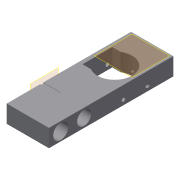
# Autodesk Inventor part: 01_Slide_camera_x_v0
Saved by Autodesk Inventor 2019.4 (Build 234330000, 330)
## iProperties
Created: 2020-10-27
Part Number: 01_Slide_camera_x_v0
Material: Generic
Document SubType Name: Modeling
Designer: diederichbenedict
Density: 1 g/cm^3
Appearance: Default
Author: diederichbenedict
Autodesk Inventor part; units mm, degrees
ref_plane "YZ Plane" through (0, 0, 0) normal (1, 0, 0) x (0, 1, 0)
ref_plane "XZ Plane" through (0, 0, 0) normal (0, 1, 0) x (-1, 0, 0)
ref_plane "XY Plane" through (0, 0, 0) normal (0, 0, 1) x (1, 0, 0)
ref_plane "Work Plane1" through (49.1675, 65.1721, -19.9847) normal (0, 1, 0) x (-1, 0, 0)
sketch "Sketch1" plane through (49.1675, 65.1721, -19.9847) normal (0, 1, 0) x (-1, 0, 0)
  circle A0 centre (-2.8102, 4.1616) radius 0.75 construction
  circle A1 centre (-2.8102, 25.1616) radius 0.75 construction
  line L0 (11.6898, 12.5705) -> (11.6898, 16.7526) construction
  arc A2 (11.6898, 16.7526) -> (11.6898, 12.5705) centre (-2.8102, 14.6616) ccw construction
  arc A3 (6.4943, 19.8433) -> (3.1979, 23.455) centre (-2.8102, 14.6616) ccw construction
  arc A4 (3.1979, 5.8681) -> (6.3691, 9.2612) centre (-2.8102, 14.6616) ccw construction
  line L1 (6.4943, 19.8433) -> (10.0762, 19.8433) construction
  line L2 (10.0762, 19.8433) -> (10.0762, 9.2612) construction
  line L3 (10.0762, 9.2612) -> (6.3691, 9.2612) construction
  arc A5 (-8.8183, 23.455) -> (-8.8183, 5.8681) centre (-2.8102, 14.6616) ccw construction
  line L4 (15.1898, -17.3384) -> (-20.8102, -17.3384)
  line L5 (-20.8102, -17.3384) -> (-20.8102, 14.6616)
  line L6 (-20.8102, 14.6616) -> (15.1898, 14.6616)
  line L7 (15.1898, 14.6616) -> (15.1898, -17.3384)
  arc A6 (4.8861, 27.3616) -> (3.5031, 1.2204) centre (-2.8102, 14.6616) ccw construction
  line L8 (4.8861, 27.3616) -> (11.8898, 27.3616) construction
  line L9 (11.8898, 27.3616) -> (11.8898, 1.9616) construction
  line L10 (11.8898, 1.9616) -> (4.7096, 1.9616) construction
  line L11 (4.7096, 1.9616) -> (2.6908, 5.7766) construction
  arc A7 (2.6908, 5.7766) -> (6.254, 9.4612) centre (-2.8102, 14.6616) ccw construction
  line L12 (6.254, 9.4612) -> (9.8762, 9.4612) construction
  line L13 (9.8762, 9.4612) -> (9.8762, 19.6433) construction
  line L14 (9.8762, 19.6433) -> (6.376, 19.6433) construction
  arc A8 (6.376, 19.6433) -> (3.2687, 23.1616) centre (-2.8102, 14.6616) ccw construction
  line L15 (3.2687, 23.1616) -> (-8.889, 23.1616) construction
  arc A9 (-8.889, 23.1616) -> (-8.446, 5.8616) centre (-2.8102, 14.6616) ccw construction
  line L16 (-8.446, 5.8616) -> (1.0472, 5.8616) construction
  line L17 (1.0472, 5.8616) -> (3.5031, 1.2204) construction
  arc A10 (-17.6602, 14.6616) -> (4.7096, 1.9616) centre (-2.9041, 14.6019) ccw
  line L18 (4.7096, 1.9616) -> (11.8943, 1.9616)
  line L19 (11.8943, 1.9616) -> (11.8898, 14.6616)
  line L20 (11.8898, 14.6616) -> (15.1898, 14.6616)
  line L21 (3.1979, 5.8681) -> (-8.8183, 5.8681) projected
  line L22 (3.1979, 23.455) -> (-8.8183, 23.455) projected
  point P0 (49.1675, 19.9847)
  dimension "d0" = 32
  dimension "d2" = 18
  dimension "d3" = 18
  dimension "d4" = 0.2
  constraints: 34 end point, 11 point on circle, 5 centre point, 2 midpoint, 2 parallel, 2 point on line, 1 collinear, 1 horizontal, 1 perpendicular, 4 other
  measures "d0" distance from line of L4 A6.centre
  measures "d2" distance from line of L7 A9.centre
  measures "d3" distance from line of L5 A6.centre
  measures "d4" radial gap between concentric circles of A2 A6
extrude "Extrusion1" add sketch "Sketch1" against normal blind 15 contours L4 L5 L6 A10 L18 L19 L7
mirror "Mirror1" about plane through (37.2777, 65.1721, -5.3231) normal (0, 0, 1) of "Extrusion1"
sketch "Sketch4" plane through (33.9777, 50.1721, -37.3231) normal (-1, 0, 0) x (0, 0, 1)
  line L0 (0, 15) -> (64, 15) projected
  line L1 (0, 15) -> (0, 0) projected
  line L2 (0, 0) -> (64, 0) projected
  line L3 (64, 15) -> (64, 0) projected
  line L4 (0, 15) -> (64, 15) projected
  line L5 (64, 15) -> (88, 15)
  line L6 (88, 15) -> (88, 0)
  line L7 (88, 0) -> (64, 0)
  line L8 (64, 0) -> (64, 15)
  circle A0 centre (56, 7.5) radius 3 projected
  circle A1 centre (56, 7.5) radius 5 projected
  circle A2 centre (76, 7.5) radius 6
  point P0 (37.3231, -50.1721)
  dimension "d20" = 24
  dimension "d21" = 12
  dimension "d24" = 12
  constraints: 8 end point, 2 parallel, 1 centre point, 1 horizontal, 1 perpendicular
  measures "d20" distance of L6.end L7.end
  measures "d21" diameter of A2
  measures "d24" distance from line of A2.centre L6
extrude "Extrusion4" add sketch "Sketch4" against normal up to surface (36 mm away) contours L5 L6 L7 L3
ref_plane "Work Plane4" through (33.9777, 57.6721, 36.6769) normal (1, 0, 0) x (0, 0, 1)
sketch "Sketch6" plane through (33.9777, 57.6721, 36.6769) normal (1, 0, 0) x (0, 0, 1)
  circle A0 centre (10, 0) radius 1.625 construction
  circle A1 centre (2, -8) radius 1.625 projected
  circle A2 centre (-6, 0) radius 1.625 construction
  circle A3 centre (2, 8) radius 1.625 projected
  circle A4 centre (2, 0) radius 4 projected
  circle A5 centre (2, 0) radius 11 construction
  line L0 (14, 7.5) -> (-74, 7.5) projected
  arc A6 (10.0467, 7.5) -> (-6.0467, 7.5) centre (2, 0) ccw
  point P0 (-36.6769, 57.6721)
  constraints: 4 point on circle, 2 point on line, 1 centre point, 1 concentric
extrude "Extrusion6" add sketch "Sketch6" along normal blind 15 contours A3 L0 | A3 L0 A6 | L0 A3
sketch "Sketch5" plane through (33.9777, 50.1721, -37.3231) normal (-1, 0, 0) x (0, 0, 1)
  circle A0 centre (68, 7.5) radius 1.625 projected
  circle A1 centre (84, 7.5) radius 1.625 projected
  circle A2 centre (84, 7.5) radius 1.45
  circle A3 centre (68, 7.5) radius 1.45
  circle A4 centre (76, 15.5) radius 1.625 projected
  circle A5 centre (76, -0.5) radius 1.625 projected
  circle A6 centre (76, -0.5) radius 1.45
  circle A7 centre (76, 15.5) radius 1.45
  point P0 (37.3231, -50.1721)
  dimension "d25" = 2.9
  dimension "d26" = 2.9
  dimension "d31" = 2.9
  dimension "d32" = 2.9
  constraints: 4 centre point, 4 coincident
  measures "d25" diameter of A2
  measures "d26" diameter of A3
  measures "d31" diameter of A6
  measures "d32" diameter of A7
extrude "Extrusion5" cut sketch "Sketch5" against normal blind 15 contours A2 | A3 | A6 | A7
sketch "Sketch7" plane through (33.9777, 50.1721, -37.3231) normal (-1, 0, 0) x (0, 0, 1)
  arc A0 (74.6389, 15) -> (77.3611, 15) centre (76, 15.5) ccw projected
  line L0 (0, 15) -> (74.6389, 15) projected
  line L1 (0, 15) -> (0, 0) projected
  line L2 (67.9533, 0) -> (0, 0) projected
  arc A1 (67.9533, 0) -> (84.0467, 0) centre (76, 7.5) ccw projected
  line L3 (88, 0) -> (84.0467, 0) projected
  line L4 (88, 15) -> (88, 0) projected
  line L5 (77.3611, 15) -> (88, 15) projected
  circle A2 centre (68, 7.5) radius 1.45 projected
  circle A3 centre (84, 7.5) radius 1.45 projected
  circle A4 centre (76, -0.5) radius 1.45 projected
  circle A5 centre (76, 7.5) radius 6 projected
  line L6 (0, 0) -> (88, 0) projected
  line L7 (88, 0) -> (106, 0)
  line L8 (106, 0) -> (106, 15)
  line L9 (106, 15) -> (88, 15)
  line L10 (88, 15) -> (88, 0)
  circle A6 centre (96, 7.5) radius 6.4305
  circle A7 centre (56, 7.5) radius 6.4532
  point P0 (37.3231, -50.1721)
  dimension "d34" = 20
  dimension "d35" = 10
  dimension "d40" = 20
  constraints: 8 end point, 2 centre point, 2 parallel, 1 horizontal, 1 perpendicular
  measures "d34" distance of A6.centre A1.centre
  measures "d35" distance from line of A6.centre L8
  measures "d40" distance of A1.centre A7.centre
extrude "Extrusion7" add sketch "Sketch7" against normal up to surface (36 mm away) contours L9 L8 L7 L4
sketch "Sketch9" plane through (33.9777, 50.1721, -37.3231) normal (-1, 0, 0) x (0, 0, 1)
  circle A0 centre (96, 7.5) radius 6.4305 projected
  circle A1 centre (56, 7.5) radius 6.4506
  point P0 (37.3231, -50.1721)
  dimension "d41" = 40
  constraints: 1 centre point
  measures "d41" distance of A0.centre A1.centre
extrude "Extrusion9" cut sketch "Sketch9" against normal through all contours A1
body "Solid1"
